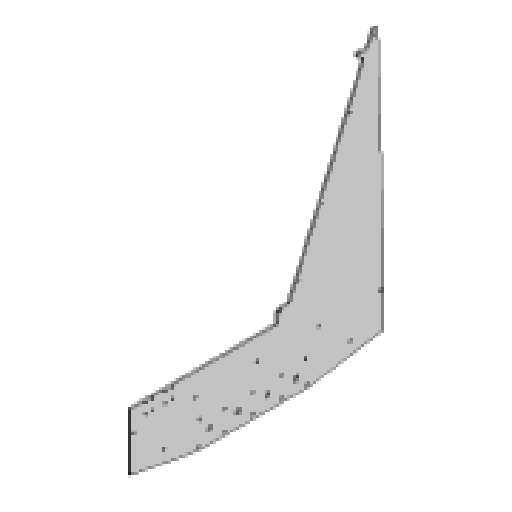
# Autodesk Inventor part: Outside Chassi Plate low 2.0
Saved by Autodesk Inventor 2023 (Build 270158000, 158)
## iProperties
Created: 2022-09-05
Part Number: Outside Chassi Plate low 2.0
Material: Generic
Document SubType Name: Modeling
Designer: deli
Density: 1 g/cm^3
Appearance: Default
Author: deli
Autodesk Inventor part; units mm, degrees
ref_plane "YZ Plane" through (0, 0, 0) normal (1, 0, 0) x (0, 1, 0)
ref_plane "XZ Plane" through (0, 0, 0) normal (0, 1, 0) x (-1, 0, 0)
ref_plane "XY Plane" through (0, 0, 0) normal (0, 0, 1) x (1, 0, 0)
sketch "Sketch1" plane through (0, 0, 0) normal (1, 0, 0) x (0, 1, 0)
  line L0 (-213.0456, 515.6134) -> (-297.8918, 515.6134)
  line L1 (-297.8918, 515.6134) -> (-316.9582, 414.9897)
  line L2 (-214.7259, 137.6134) -> (-299.5721, 137.6134)
  circle A0 centre (-289.0456, 465.6134) radius 2
  circle A1 centre (-289.0456, 465.6134) radius 48 construction
  arc A2 (-277.1614, 464.4968) -> (-300.901, 467.0036) centre (-289.0456, 465.6134) ccw construction
  circle A3 centre (-289.0456, 187.6134) radius 48 construction
  arc A4 (-300.924, 186.4354) -> (-277.1466, 188.5592) centre (-289.0456, 187.6134) ccw construction
  circle A5 centre (-289.0456, 187.6134) radius 2
  circle A6 centre (-296.2956, 396.9562) radius 4
  circle A7 centre (-296.2956, 268.785) radius 4
  circle A8 centre (-296.2956, 396.9562) radius 18.75 construction
  circle A9 centre (-296.2956, 268.785) radius 18.75 construction
  arc A10 (-308.9414, 398.4391) -> (-283.6191, 395.7651) centre (-296.2956, 396.9562) ccw construction
  arc A11 (-283.6033, 269.7939) -> (-308.9659, 267.5285) centre (-296.2956, 268.785) ccw construction
  line L3 (-277.1614, 464.4968) -> (-283.6191, 395.7651) construction
  line L4 (-308.9414, 398.4391) -> (-300.901, 467.0036) construction
  line L5 (-283.6033, 269.7939) -> (-277.1466, 188.5592) construction
  line L6 (-300.924, 186.4354) -> (-308.9659, 267.5285) construction
  circle A12 centre (-281.8153, 290.0778) radius 2
  circle A13 centre (-310.776, 290.0778) radius 2
  circle A14 centre (-312.0456, 251.6824) radius 2
  circle A15 centre (-278.3368, 254.0187) radius 2
  circle A16 centre (-246.0456, 510.6134) radius 2
  arc A17 (-317.0456, 229.9036) -> (-317.0456, 229.9036) centre (-294.2956, 229.9036) ccw
  line L7 (-317.0456, 251.6824) -> (-317.0456, 229.9036)
  arc A18 (-316.9582, 414.9897) -> (-317.0456, 414.0588) centre (-312.0456, 414.0588) ccw
  line L8 (-317.0456, 414.0588) -> (-317.0456, 229.9036)
  line L9 (-299.5721, 137.6134) -> (-316.9876, 250.9228)
  circle A19 centre (-278.1266, 411.463) radius 2
  arc A20 (-317.0456, 251.6824) -> (-316.9876, 250.9228) centre (-312.0456, 251.6824) ccw
  circle A21 centre (-246.0456, 234.6134) radius 2
  line L10 (-213.0456, 515.6134) -> (-213.0456, 295.3514)
  circle A22 centre (-246.0456, 418.6134) radius 2
  circle A23 centre (-246.0456, 326.6134) radius 2
  circle A24 centre (-312.0456, 414.0588) radius 2
  circle A25 centre (-246.0456, 142.6134) radius 2
  line L11 (-178.803, 271.1115) -> (-181.565, 264.6795)
  line L12 (-181.565, 264.6795) -> (94.0945, 146.3078)
  line L13 (94.0945, 146.3078) -> (96.8565, 152.7399)
  line L14 (628.6384, -183.2052) -> (619.1262, -197.2948) construction
  line L15 (-182.3379, 275.5515) -> (-189.0456, 259.9308) construction
  line L16 (-188.4024, 278.1557) -> (108.5747, 150.6299) construction
  line L17 (102.5102, 153.2341) -> (95.8025, 137.6134) construction
  line L18 (95.8025, 137.6134) -> (-189.0456, 259.9308) construction
  line L19 (-184.6634, 282.8078) -> (-173.6371, 278.073) construction
  line L20 (-173.6371, 278.073) -> (-175.2154, 274.3975) construction
  line L21 (-175.2154, 274.3975) -> (-186.2417, 279.1324) construction
  line L22 (-186.2417, 279.1324) -> (-184.6634, 282.8078) construction
  line L23 (-185.4431, 285.0472) -> (-176.0707, 281.0225) construction
  line L24 (-178.4381, 275.5093) -> (-187.8106, 279.534) construction
  line L25 (-176.0707, 281.0225) -> (-176.6626, 279.6442) construction
  line L26 (-178.4381, 275.5093) -> (-179.03, 274.131) construction
  line L27 (-176.6626, 279.6442) -> (-186.035, 283.6689) construction
  arc A26 (-185.4431, 285.0472) -> (-188.4024, 278.1557) centre (-186.9228, 281.6014) ccw construction
  arc A27 (-186.035, 283.6689) -> (-187.8106, 279.534) centre (-186.9228, 281.6014) ccw construction
  line L28 (99.2023, 154.6546) -> (99.7941, 156.0328) construction
  line L29 (99.7941, 156.0328) -> (109.1666, 152.0082) construction
  arc A28 (109.1666, 152.0082) -> (110.9421, 156.1431) centre (110.0544, 154.0757) ccw construction
  line L30 (110.9421, 156.1431) -> (101.5697, 160.1677) construction
  line L31 (101.5697, 160.1677) -> (102.1616, 161.546) construction
  line L32 (102.1616, 161.546) -> (111.534, 157.5214) construction
  arc A29 (108.5747, 150.6299) -> (111.534, 157.5214) centre (110.0544, 154.0757) ccw construction
  line L33 (109.3733, 156.5447) -> (107.795, 152.8692) construction
  line L34 (107.795, 152.8692) -> (96.7686, 157.6041) construction
  line L35 (96.7686, 157.6041) -> (98.3469, 161.2796) construction
  line L36 (98.3469, 161.2796) -> (109.3733, 156.5447) construction
  line L37 (94.0945, 146.3078) -> (-214.7259, 137.6134)
  circle A30 centre (-173.2925, 264.9362) radius 1
  circle A31 centre (-90.5947, 229.4247) radius 1
  circle A32 centre (5.8861, 187.9946) radius 1
  circle A33 centre (88.584, 152.4831) radius 1
  circle A34 centre (73.8024, 175.0842) radius 1.5
  arc A35 (76.559, 173.9005) -> (71.0458, 176.2679) centre (73.8024, 175.0842) ccw
  line L38 (71.0458, 176.2679) -> (68.4131, 170.1368)
  line L39 (76.559, 173.9005) -> (73.9263, 167.7694)
  line L40 (96.8565, 152.7399) -> (76.4232, 161.5142)
  line L41 (62.1578, 167.6399) -> (-195.0456, 278.0863)
  arc A36 (73.9263, 167.7694) -> (76.4232, 161.5142) centre (78.3024, 165.8902) ccw
  arc A37 (62.1578, 167.6399) -> (68.4131, 170.1368) centre (64.037, 172.016) ccw
  circle A38 centre (73.8024, 175.0842) radius 6 construction
  circle A39 centre (-215.5456, 490.1634) radius 1.6
  circle A40 centre (-230.5456, 490.1634) radius 1.6
  circle A41 centre (-230.5456, 480.1634) radius 1.6
  circle A42 centre (-215.5456, 480.1634) radius 1.6
  circle A43 centre (-215.5456, 461.2634) radius 1.6
  circle A44 centre (-215.5456, 451.2634) radius 1.6
  circle A45 centre (-230.5456, 451.2634) radius 1.6
  circle A46 centre (-230.5456, 461.2634) radius 1.6
  line L42 (-215.5456, 490.1634) -> (-230.5456, 490.1634) construction
  line L43 (-230.5456, 490.1634) -> (-230.5456, 480.1634) construction
  line L44 (-230.5456, 480.1634) -> (-215.5456, 480.1634) construction
  line L45 (-215.5456, 480.1634) -> (-215.5456, 490.1634) construction
  line L46 (-215.5456, 451.2634) -> (-215.5456, 461.2634) construction
  line L47 (-215.5456, 461.2634) -> (-230.5456, 461.2634) construction
  line L48 (-230.5456, 461.2634) -> (-230.5456, 451.2634) construction
  line L49 (-230.5456, 451.2634) -> (-215.5456, 451.2634) construction
  line L50 (-296.2956, 396.9562) -> (-296.2956, 268.785) construction
  circle A47 centre (-296.2956, 354.3706) radius 18.75 construction
  circle A48 centre (-296.2956, 311.3706) radius 18.75 construction
  line L51 (-241.0456, 515.6134) -> (-241.0456, 137.6134) construction
  circle A49 centre (-296.2956, 354.3706) radius 4
  circle A50 centre (-296.2956, 311.3706) radius 4
  circle A51 centre (-282.1248, 332.8706) radius 2
  circle A52 centre (-310.4665, 332.8706) radius 2
  circle A53 centre (-281.8153, 375.6634) radius 2
  circle A54 centre (-310.776, 375.6634) radius 2
  circle A55 centre (-198.0456, 292.3514) radius 2
  arc A56 (-195.0456, 292.3514) -> (-198.0456, 295.3514) centre (-198.0456, 292.3514) ccw
  line L52 (-195.0456, 292.3514) -> (-195.0456, 278.0863)
  line L53 (-198.0456, 295.3514) -> (-213.0456, 295.3514)
  point P0 (0, 0)
  point P1 (-317.0456, 251.6824)
  point P2 (-225.2933, 137.6134)
  dimension "d44" = 4
  dimension "d46" = 96
  dimension "d47" = 23.8732
  dimension "d51" = 23.8732
  dimension "d54" = 50
  dimension "d55" = 50
  dimension "d58" = 8
  dimension "d60" = 37.5
  dimension "d62" = 25.4648
  dimension "d64" = 178.679
  dimension "d65" = 178.679
  dimension "d66" = 178.881
  dimension "d67" = 178.881
  dimension "d68" = 69.0344
  dimension "d70" = 81.4909
  dimension "d94" = 2.5
  dimension "d95" = 2.5
  dimension "d103" = 4
  dimension "d124" = 28
  dimension "d142" = 4
  dimension "d143" = 2.5
  dimension "d144" = 4
  dimension "d145" = 4
  dimension "d146" = 18
  dimension "d147" = 18
  dimension "d148" = 5
  dimension "d149" = 5
  dimension "d153" = 4
  dimension "d218" = 0
  dimension "d235" = 33
  dimension "d244" = 28
  dimension "d246" = 84.8462
  dimension "d247" = 84.8462
  dimension "d258" = 5
  dimension "d259" = 5
  dimension "d260" = 4
  dimension "d261" = 4
  dimension "d266" = 33
  dimension "d267" = 33
  dimension "d268" = 92
  dimension "d269" = 92
  dimension "d270" = 92
  dimension "d277" = 5
  dimension "d296" = 33
  dimension "d297" = 7
  dimension "d317" = 0
  dimension "d333" = 378
  dimension "d334" = 5
  dimension "d336" = 17
  dimension "d338" = 5
  dimension "d339" = 5
  dimension "d340" = 300
  dimension "d342" = 4
  dimension "d343" = 12
  dimension "d344" = 7
  dimension "d345" = 6.6
  dimension "d346" = 2
  dimension "d347" = 10.2
  dimension "d348" = 1.5
  dimension "d349" = 1.5
  dimension "d350" = 3.75
  dimension "d351" = 1.5
  dimension "d353" = 3.75
  dimension "d354" = 6.6
  constraints: 108 end point, 57 centre point, 31 point on circle, 30 equal radius, 28 tangent, 25 perpendicular, 15 parallel, 14 coincident, 11 point on line, 6 vertical, 4 collinear, 4 concentric, 3 equal length
  measures "d44" diameter of A0
  measures "d46" diameter of A1
  measures "d47" diameter of A2
  measures "d51" diameter of A4
  measures "d54" distance from line of A0.centre L0
  measures "d55" distance from line of L2 A5.centre
  measures "d58" diameter of A6
  measures "d60" diameter of A8
  measures "d62" diameter of A10
  measures "d68" distance of L3.start L3.end
  measures "d70" distance of L5.start L5.end
  measures "d103" diameter of A16
  measures "d124" distance from line of A0.centre L7
  measures "d142" distance from line of L5 A15.centre
  measures "d144" distance from line of L3 A19.centre
  measures "d145" diameter of A19
  measures "d146" distance from line of A0.centre L1
  measures "d147" distance from line of L9 A3.centre
  measures "d148" radius of A18
  measures "d149" radius of A20
  measures "d153" diameter of A21
  measures "d218" horizontal distance of A0.centre A5.centre
  measures "d235" distance from line of L10 A16.centre
  measures "d244" distance edge to line of A1 L10
  measures "d246" distance of L2.start L2.end
  measures "d247" distance of L0.start L0.end
  measures "d260" diameter of A22
  measures "d261" diameter of A23
  measures "d266" distance from line of L10 A22.centre
  measures "d267" distance from line of L10 A23.centre
  measures "d268" distance of A22.centre A16.centre
  measures "d269" distance of A23.centre A22.centre
  measures "d270" distance of A21.centre A23.centre
  measures "d277" distance from line of L2 A25.centre
  measures "d296" distance from line of L10 A21.centre
  measures "d297" distance of L11.start L11.end
  measures "d317" horizontal distance of A25.centre A21.centre
  measures "d333" distance between parallel lines of L2 L0
  measures "d334" distance from line of L0 A16.centre
  measures "d336" distance between parallel lines of L18 L16
  measures "d338" distance between parallel lines of L11 L15
  measures "d339" distance between parallel lines of L13 L17
  measures "d340" distance of L11.end L12.end
  measures "d342" distance of L19.end L20.end
  measures "d343" distance of L19.start L19.end
  measures "d344" distance between parallel lines of L15 L20
  measures "d345" distance from line of L15 A26.centre
  measures "d346" distance from line of A26.centre L21
  measures "d347" distance of L23.start L23.end
  measures "d348" distance of L24.start L26.end
  measures "d349" distance of L23.end L25.end
  measures "d350" radius of A26
  measures "d351" distance of L28.start L28.end
  measures "d353" radius of A29
  measures "d354" distance from line of L17 A28.centre
extrude "Extrusion1" add sketch "Sketch1" along normal blind 3.175 contours L10 L53 A56 L52 L41 L11 L12 L37 L2 L9 A17 A20 L8 A18 L1 L0 | L41 A37 L38 A35 L39 A36 L40 L13 L12 L11 | A17 L9 picked at (-288.2245, 226.0657)
thread "Thread1" size "M2x0.4" class "6H" standard "ANSI Metric M Profile" full length
thread "Thread2" size "M2x0.4" class "6H" standard "ANSI Metric M Profile" full length
thread "Thread3" size "M2x0.4" class "6H" standard "ANSI Metric M Profile" full length
fillet "Fillet1" radius 2 3 edges at (1.5875, 96.8565, 152.7399) (1.5875, -195.0456, 278.0863) (1.5875, -213.0456, 295.3514)
thread "Thread4" size "M2x0.4" class "6H" standard "ANSI Metric M Profile" full length
body "Solid1"
